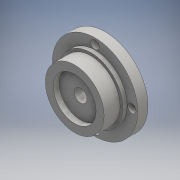
# Autodesk Inventor part: GearHead2
Saved by Autodesk Inventor 2016 (Build 200138000, 138)
## iProperties
Created: 2016-06-23
Part Number: GearHead2
Material: 一般
Document SubType Name: Modeling
Designer: 宏太
Density: 1 g/cm^3
Appearance: 既定
Mass: 84.3972 g
Surface Area: 178.024 cm^2
Volume: 84.3972 cm^3
Author: 宏太
Autodesk Inventor part; units mm, degrees
ref_plane "YZ Plane" through (0, 0, 0) normal (1, 0, 0) x (0, 1, 0)
ref_plane "XZ Plane" through (0, 0, 0) normal (0, 1, 0) x (-1, 0, 0)
ref_plane "XY Plane" through (0, 0, 0) normal (0, 0, 1) x (1, 0, 0)
sketch "スケッチ1" plane through (0, 0, 0) normal (0, 1, 0) x (-1, 0, 0)
  circle A0 centre (0, 0) radius 40
  dimension "d0" = 80
  constraints: 1 centre point, 1 coincident
  measures "d0" diameter of A0
extrude "押し出し1" add sketch "スケッチ1" along normal blind 28.6
sketch "スケッチ2" plane through (0, 0, 0) normal (0, -1, 0) x (1, 0, 0)
  circle A0 centre (0, 0) radius 30.05
  circle A1 centre (0, 0) radius 40
  dimension "d3" = 60.1
  dimension "d4" = 80
  constraints: 2 centre point, 2 coincident
  measures "d3" diameter of A0
  measures "d4" diameter of A1
extrude "押し出し2" cut sketch "スケッチ2" against normal blind 19
sketch "スケッチ3" plane through (0, 0, 0) normal (0, -1, 0) x (1, 0, 0)
  circle A0 centre (0, 0) radius 27.5
  circle A1 centre (0, 0) radius 30.05
  dimension "d7" = 55
  constraints: 2 centre point, 2 coincident
  measures "d7" diameter of A0
extrude "押し出し3" cut sketch "スケッチ3" against normal blind 15
sketch "スケッチ5" plane through (0, 0, 0) normal (0, -1, 0) x (1, 0, 0)
  circle A0 centre (0, 0) radius 20
  dimension "d10" = 40
  constraints: 1 centre point, 1 coincident
  measures "d10" diameter of A0
extrude "押し出し4" cut sketch "スケッチ5" against normal blind 5.5
sketch "スケッチ6" plane through (0, 5.5, 0) normal (0, -1, 0) x (1, 0, 0)
  circle A0 centre (0, 0) radius 6
  dimension "d13" = 12
  constraints: 1 centre point, 1 coincident
  measures "d13" diameter of A0
extrude "押し出し5" cut sketch "スケッチ6" against normal blind 30000
sketch "スケッチ7" plane through (0, 19, 0) normal (0, -1, 0) x (1, 0, 0)
  circle A0 centre (0, 0) radius 34.5
  circle A1 centre (0, 34.5) radius 2
  circle A2 centre (34.5, 0) radius 2
  circle A3 centre (0, -34.5) radius 2
  circle A4 centre (-34.4997, 0.1397) radius 2
  dimension "d60" = 69
  dimension "d61" = 4
  dimension "d62" = 4
  dimension "d63" = 4
  dimension "d64" = 4
  constraints: 5 centre point, 4 point on circle, 1 coincident
  measures "d60" diameter of A0
  measures "d61" diameter of A1
  measures "d62" diameter of A2
  measures "d63" diameter of A3
  measures "d64" diameter of A4
extrude "押し出し6" cut sketch "スケッチ7" against normal blind 10 contours A0 A2 | A0 A2 | A1 A0 | A0 A1 | A3 A0 | A0 A3 | A4 A0 | A0 A4
hole "穴1" at (34.5, 19, 0) direction (0, 1, 0) diameter 4.2 depth 10 counterbore diameter 8 counterbore depth 5.4
hole "穴2" at (-34.4997, 19, 0.1397) direction (0, 1, 0) diameter 4.2 depth 10 counterbore diameter 8 counterbore depth 5.4
hole "穴3" at (0, 19, -34.5) direction (0, 1, 0) diameter 4.2 depth 10 counterbore diameter 8 counterbore depth 5.4
hole "穴4" at (0, 19, 34.5) direction (0, 1, 0) diameter 4.2 depth 10 counterbore diameter 8 counterbore depth 5.4
